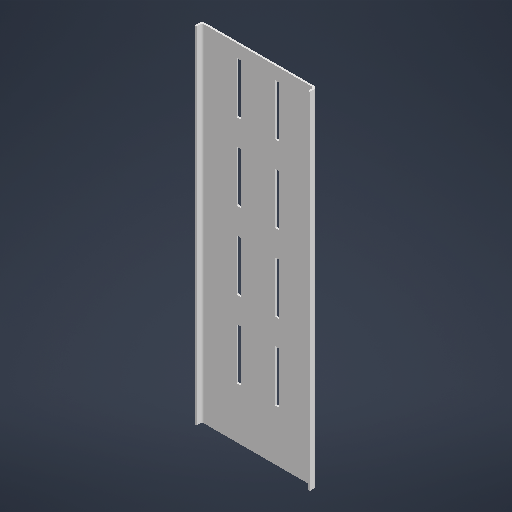
# Autodesk Inventor part: TrayRail
Saved by Autodesk Inventor 2026.3 (Build 303398000, 398)
## iProperties
Created: 2026-05-01
Part Number: TrayRail
Material: Generic
Document SubType Name: Sheet Metal
Designer: frede
Density: 1 g/cm^3
Sheet Metal Rule: Default_mm
Appearance: Default
Author: frede
Autodesk Inventor part; units mm, degrees
ref_plane "YZ Plane" through (0, 0, 0) normal (1, 0, 0) x (0, 1, 0)
ref_plane "XZ Plane" through (0, 0, 0) normal (0, 1, 0) x (-1, 0, 0)
ref_plane "XY Plane" through (0, 0, 0) normal (0, 0, 1) x (1, 0, 0)
sketch "Sketch1" plane through (0, 0, 0) normal (0, 0, 1) x (1, 0, 0)
  line L0 (61, -189) -> (-61, -189)
  line L1 (-61, -189) -> (-61, 189)
  line L2 (-61, 189) -> (61, 189)
  line L3 (61, 189) -> (61, -189)
  line L4 (61, -189) -> (-61, 189) construction
  line L5 (-61, -189) -> (61, 189) construction
  point P0 (0, 0)
  dimension "d0" = 122
  dimension "d1" = 378
  measures "d0" distance of L1.end L2.end
  measures "d1" distance between parallel lines of L0 L2
extrude "Plate1" add sketch "Sketch1" along normal blind 2
sketch "Sketch3" plane through (-63, -189, 0) normal (1, 0, 0) x (0, 1, 0)
  line L0 (378, 0) -> (0, 0)
  line L1 (0, 0) -> (0, 8)
  line L2 (0, 8) -> (378, 8)
  line L3 (378, 8) -> (378, 0)
  constraints: 8 end point
edge flange "Flange1" height 8 angle 90 thickness 2 bend radius 2 thickness toward (1, 0, 0) relief tear relief width 2 relief depth 1 corner gap 2 corner form 0 edges at (-61, 0, 2) (61, 0, 2) wall of the first edge with corners at (-63, 189, 0) (-63, -189, 0) (-63, -189, 8) (-63, 189, 8)
bend "Bend1"
corner "Corner1"
sketch "Sketch4" plane through (0, 0, 2) normal (0, 0, 1) x (1, 0, 0)
  line L0 (59, -189) -> (-59, -189) projected
  line L1 (-59, 189) -> (59, 189) projected
  line L2 (60.25, 63) -> (-60.25, 63)
  line L3 (-60.25, 63) -> (-60.25, 189)
  line L4 (-60.25, 189) -> (60.25, 189)
  line L5 (60.25, 189) -> (60.25, 63)
  line L6 (60.25, 63) -> (-60.25, 189) construction
  line L7 (-60.25, 63) -> (60.25, 189) construction
  line L8 (-21, 189) -> (-21, -189)
  line L9 (21, 189) -> (21, -189)
  line L10 (-23.25, 174.5) -> (-23.25, 119.5)
  line L11 (-18.75, 174.5) -> (-18.75, 119.5)
  line L12 (18.75, 174.5) -> (18.75, 119.5)
  line L13 (23.25, 174.5) -> (23.25, 119.5)
  line L14 (-22.75, 175) -> (-19.25, 175)
  line L15 (19.25, 175) -> (22.75, 175)
  line L16 (-22.75, 119) -> (-19.25, 119)
  line L17 (19.25, 119) -> (22.75, 119)
  arc A0 (-22.75, 175) -> (-23.25, 174.5) centre (-22.75, 174.5) ccw
  arc A1 (-18.75, 174.5) -> (-19.25, 175) centre (-19.25, 174.5) ccw
  arc A2 (-19.25, 119) -> (-18.75, 119.5) centre (-19.25, 119.5) ccw
  arc A3 (-23.25, 119.5) -> (-22.75, 119) centre (-22.75, 119.5) ccw
  arc A4 (18.75, 119.5) -> (19.25, 119) centre (19.25, 119.5) ccw
  arc A5 (22.75, 119) -> (23.25, 119.5) centre (22.75, 119.5) ccw
  arc A6 (19.25, 175) -> (18.75, 174.5) centre (19.25, 174.5) ccw
  arc A7 (23.25, 174.5) -> (22.75, 175) centre (22.75, 174.5) ccw
  line L18 (-22.75, 91) -> (-19.25, 91)
  arc A8 (-18.75, 90.5) -> (-19.25, 91) centre (-19.25, 90.5) ccw
  line L19 (-18.75, 90.5) -> (-18.75, 35.5)
  arc A9 (-22.75, 91) -> (-23.25, 90.5) centre (-22.75, 90.5) ccw
  line L20 (-23.25, 90.5) -> (-23.25, 35.5)
  line L21 (-22.75, 35) -> (-19.25, 35)
  arc A10 (-23.25, 35.5) -> (-22.75, 35) centre (-22.75, 35.5) ccw
  arc A11 (-19.25, 35) -> (-18.75, 35.5) centre (-19.25, 35.5) ccw
  line L22 (19.25, 35) -> (22.75, 35)
  arc A12 (22.75, 35) -> (23.25, 35.5) centre (22.75, 35.5) ccw
  arc A13 (18.75, 35.5) -> (19.25, 35) centre (19.25, 35.5) ccw
  line L23 (18.75, 90.5) -> (18.75, 35.5)
  line L24 (23.25, 90.5) -> (23.25, 35.5)
  line L25 (19.25, 91) -> (22.75, 91)
  arc A14 (23.25, 90.5) -> (22.75, 91) centre (22.75, 90.5) ccw
  arc A15 (19.25, 91) -> (18.75, 90.5) centre (19.25, 90.5) ccw
  line L26 (-22.75, 7) -> (-19.25, 7)
  arc A16 (-18.75, 6.5) -> (-19.25, 7) centre (-19.25, 6.5) ccw
  line L27 (-18.75, 6.5) -> (-18.75, -48.5)
  arc A17 (-22.75, 7) -> (-23.25, 6.5) centre (-22.75, 6.5) ccw
  line L28 (-23.25, 6.5) -> (-23.25, -48.5)
  line L29 (-22.75, -49) -> (-19.25, -49)
  arc A18 (-23.25, -48.5) -> (-22.75, -49) centre (-22.75, -48.5) ccw
  arc A19 (-19.25, -49) -> (-18.75, -48.5) centre (-19.25, -48.5) ccw
  line L30 (19.25, -49) -> (22.75, -49)
  arc A20 (22.75, -49) -> (23.25, -48.5) centre (22.75, -48.5) ccw
  arc A21 (18.75, -48.5) -> (19.25, -49) centre (19.25, -48.5) ccw
  line L31 (18.75, 6.5) -> (18.75, -48.5)
  line L32 (23.25, 6.5) -> (23.25, -48.5)
  line L33 (19.25, 7) -> (22.75, 7)
  arc A22 (23.25, 6.5) -> (22.75, 7) centre (22.75, 6.5) ccw
  arc A23 (19.25, 7) -> (18.75, 6.5) centre (19.25, 6.5) ccw
  line L34 (-22.75, -77) -> (-19.25, -77)
  arc A24 (-18.75, -77.5) -> (-19.25, -77) centre (-19.25, -77.5) ccw
  line L35 (-18.75, -77.5) -> (-18.75, -132.5)
  arc A25 (-22.75, -77) -> (-23.25, -77.5) centre (-22.75, -77.5) ccw
  line L36 (-23.25, -77.5) -> (-23.25, -132.5)
  line L37 (-22.75, -133) -> (-19.25, -133)
  arc A26 (-23.25, -132.5) -> (-22.75, -133) centre (-22.75, -132.5) ccw
  arc A27 (-19.25, -133) -> (-18.75, -132.5) centre (-19.25, -132.5) ccw
  line L38 (19.25, -133) -> (22.75, -133)
  arc A28 (22.75, -133) -> (23.25, -132.5) centre (22.75, -132.5) ccw
  arc A29 (18.75, -132.5) -> (19.25, -133) centre (19.25, -132.5) ccw
  line L39 (18.75, -77.5) -> (18.75, -132.5)
  line L40 (23.25, -77.5) -> (23.25, -132.5)
  line L41 (19.25, -77) -> (22.75, -77)
  arc A30 (23.25, -77.5) -> (22.75, -77) centre (22.75, -77.5) ccw
  arc A31 (19.25, -77) -> (18.75, -77.5) centre (19.25, -77.5) ccw
  line L42 (60.25, -63) -> (-60.25, -63)
  point P0 (0, 0)
  point P1 (0, 126)
  dimension "d17" = 120.5
  dimension "d18" = 60.25
  dimension "d19" = 21
  dimension "d20" = 42
  dimension "d22" = 4.5
  dimension "d23" = 2.25
  dimension "d24" = 4.5
  dimension "d25" = 2.25
  dimension "d26" = 56
  dimension "d27" = 56
  dimension "d28" = 0.5
  dimension "d31" = 84
  dimension "d38" = 126
  constraints: 82 end point, 64 point on circle, 32 centre point, 16 tangent, 7 equal radius, 7 perpendicular, 5 point on line, 4 vertical, 3 horizontal, 2 midpoint, 2 parallel, 123 other
  measures "d17" distance of L3.end L4.end
  measures "d18" distance from line of L3 point (0, 0)
  measures "d19" distance from line of point (0, 0) L8
  measures "d20" distance between parallel lines of L9 L8
  measures "d22" distance between parallel lines of L11 L10
  measures "d23" distance between parallel lines of L8 L10
  measures "d24" distance between parallel lines of L13 L12
  measures "d25" distance between parallel lines of L13 L9
  measures "d26" distance between parallel lines of L16 L14
  measures "d27" distance between parallel lines of L17 L15
  measures "d28" radius of A0
  measures "d31" distance of L14.start L18.start
  measures "d38" distance of L2.start L42.start
extrude "Extrusion2" cut sketch "Sketch4" against normal blind 2 contours L38 A29 L39 A31 L41 L9 | L9 L41 A30 L40 A28 L38 | L37 A26 L36 A25 L34 L8 | L8 L34 A24 L35 A27 L37 | L30 A21 L31 A23 L33 L9 | L9 L33 A22 L32 A20 L30 | L29 A18 L28 A17 L26 L8 | L8 L26 A16 L27 A19 L29 | L22 A13 L23 L2 L9 | L9 L2 L24 A12 L22 | L21 A10 L20 L2 L8 | L8 L2 L19 A11 L21 | L9 L25 A14 L24 L2 | L2 L23 A15 L25 L9 | L8 L18 A8 L19 L2 | L2 L20 A9 L18 L8 | L17 A4 L12 A6 L15 L9 | L9 L15 A7 L13 A5 L17 | L16 A3 L10 A0 L14 L8 | L8 L14 A1 L11 A2 L16
equation "\"d18\" = 0.5 * d17"
equation "\"d19\" = 0.5 * d20"
equation "\"d23\" = 0.5 * d22"
equation "\"d25\" = 0.5 * d24"
equation "\"d27\" = d26"
equation "\"d4\" = Thickness"
equation "\"d5\" = BendReliefWidth"
equation "\"d6\" = BendReliefDepth"
equation "\"d7\" = MinimumRemnant"
equation "\"d8\" = TransitionRadius"
equation "\"d11\" = BendRadius"
equation "\"d12\" = CornerReliefSize"
equation "\"d13\" = GapSize"
equation "\"d14\" = JacobiRadiusSize"
equation "\"BendRadius\" = Thickness"
equation "\"BendReliefWidth\" = Thickness"
equation "\"BendReliefDepth\" = 0.5 * Thickness"
equation "\"CornerReliefSize\" = 4 * Thickness"
equation "\"MinimumRemnant\" = 2 * Thickness"
equation "\"TransitionRadius\" = BendRadius"
equation "\"JacobiRadiusSize\" = BendRadius"
equation "\"GapSize\" = Thickness"
equation "\"Thickness\" = 2"
body "Solid2"
